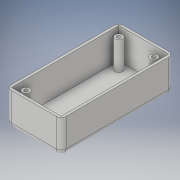
# Autodesk Inventor part: BottomcaseV2
Saved by Autodesk Inventor 2019 (Build 230136000, 136)
## iProperties
Created: 2019-05-05
Part Number: BottomcaseV2
Material: Generic
Document SubType Name: Modeling
Designer: Henry
Density: 1 g/cm^3
Appearance: Default
Author: Henry
Autodesk Inventor part; units mm, degrees
ref_plane "YZ Plane" through (0, 0, 0) normal (1, 0, 0) x (0, 1, 0)
ref_plane "XZ Plane" through (0, 0, 0) normal (0, 1, 0) x (-1, 0, 0)
ref_plane "XY Plane" through (0, 0, 0) normal (0, 0, 1) x (1, 0, 0)
sketch "Sketch1" plane through (0, 0, 0) normal (0, 1, 0) x (-1, 0, 0)
  line L0 (0, 0) -> (40.5, 0)
  line L1 (40.5, 0) -> (40.5, -87.5)
  line L2 (40.5, -87.5) -> (0, -87.5)
  line L3 (0, -87.5) -> (0, 0)
  dimension "d0" = 40.5
  dimension "d1" = 87.5
  constraints: 8 end point, 2 parallel, 1 horizontal, 1 perpendicular
  measures "d0" distance of L1.end L2.end
  measures "d1" distance of L0.end L1.end
extrude "Extrusion1" add sketch "Sketch1" along normal blind 2
sketch "Sketch3" plane through (0, 2, 0) normal (0, 1, 0) x (1, 0, 0)
  line L0 (-40.5, 0) -> (0, 0) projected
  line L1 (-40.5, 0) -> (-34.5, 0)
  line L2 (-34.5, 0) -> (-34.5, 6)
  line L3 (-34.5, 6) -> (-40.5, 6)
  line L4 (-40.5, 6) -> (-40.5, 0)
  circle A0 centre (-34.5, 6) radius 3
  line L5 (-40.5, 87.5) -> (-40.5, 0) projected
  line L6 (-40.5, 87.5) -> (-34.5, 87.5)
  line L7 (-34.5, 87.5) -> (-34.5, 81.5)
  line L8 (-34.5, 81.5) -> (-40.5, 81.5)
  line L9 (-40.5, 81.5) -> (-40.5, 87.5)
  circle A1 centre (-34.5, 81.5) radius 3
  line L10 (0, 0) -> (0, 87.5) projected
  line L11 (0, 87.5) -> (-6, 87.5)
  line L12 (-6, 87.5) -> (-6, 81.5)
  line L13 (-6, 81.5) -> (0, 81.5)
  line L14 (0, 81.5) -> (0, 87.5)
  circle A2 centre (-6, 81.5) radius 3
  dimension "d4" = 6
  dimension "d5" = 6
  dimension "d6" = 6
  dimension "d7" = 6
  dimension "d8" = 6
  dimension "d9" = 6
  dimension "d10" = 6
  dimension "d11" = 6
  dimension "d12" = 6
  constraints: 24 end point, 6 parallel, 3 centre point, 3 coincident, 3 horizontal, 3 perpendicular
  measures "d4" distance of L3.end L2.end
  measures "d5" distance of L2.end L1.end
  measures "d6" diameter of A0
  measures "d7" distance of L7.end L8.end
  measures "d8" distance of L6.end L7.end
  measures "d9" diameter of A1
  measures "d10" distance of L13.end L12.end
  measures "d11" distance of L12.end L11.end
  measures "d12" diameter of A2
extrude "Extrusion2" add sketch "Sketch3" along normal blind 23 contours A0 L3 L2 | L2 L3 A0 | A1 L7 L8 | L8 L7 A1 | A2 L12 L13 | L13 L12 A2
sketch "Sketch4" plane through (-34.5, 25, -6) normal (0, 1, 0) x (1, 0, 0)
  circle A0 centre (0, 0) radius 1.5
  point P0 (34.5, -6)
  dimension "d15" = 3
  constraints: 1 centre point
  measures "d15" diameter of A0
sketch "Sketch5" plane through (-34.5, 25, -81.5) normal (0, 1, 0) x (1, 0, 0)
  circle A0 centre (0, 0) radius 1.5
  point P0 (34.5, -81.5)
  dimension "d16" = 3
  constraints: 1 centre point
  measures "d16" diameter of A0
sketch "Sketch6" plane through (-6, 25, -81.5) normal (0, 1, 0) x (1, 0, 0)
  circle A0 centre (0, 0) radius 1.5
  point P0 (6, -81.5)
  dimension "d17" = 3
  constraints: 1 centre point
  measures "d17" diameter of A0
extrude "Extrusion3" cut sketch "Sketch4" against normal blind 12
extrude "Extrusion4" cut sketch "Sketch5" against normal blind 12
extrude "Extrusion5" cut sketch "Sketch6" against normal blind 12
sketch "Sketch7" plane through (0, 0, 0) normal (0, -1, 0) x (1, 0, 0)
  line L0 (0, 0) -> (0, -87.5) projected
  line L1 (0, 0) -> (2, 0)
  line L2 (2, 0) -> (2, -87.5)
  line L3 (2, -87.5) -> (0, -87.5)
  line L4 (0, -87.5) -> (0, 0)
  line L5 (-40.5, 0) -> (0, 0) projected
  line L6 (-40.5, 0) -> (-42.5, 0)
  line L7 (-42.5, 0) -> (-42.5, -87.5)
  line L8 (-42.5, -87.5) -> (-40.5, -87.5)
  line L9 (-40.5, -87.5) -> (-40.5, 0)
  line L10 (-42.5, -87.5) -> (2, -87.5)
  line L11 (2, -87.5) -> (2, -89.5)
  line L12 (2, -89.5) -> (-42.5, -89.5)
  line L13 (-42.5, -89.5) -> (-42.5, -87.5)
  line L14 (-42.5, 0) -> (2, 0)
  line L15 (2, 0) -> (2, 2)
  line L16 (2, 2) -> (-42.5, 2)
  line L17 (-42.5, 2) -> (-42.5, 0)
  dimension "d24" = 2
  dimension "d25" = 2
  dimension "d26" = 2
  dimension "d27" = 2
  constraints: 32 end point, 8 parallel, 4 horizontal, 4 perpendicular, 1 point on line
  measures "d24" distance of L2.end L3.end
  measures "d25" distance of L8.end L7.end
  measures "d26" distance of L10.end L11.end
  measures "d27" distance of L15.end L14.end
extrude "Extrusion6" add sketch "Sketch7" against normal blind 27 contours L1 L2 L3 L0 | L5 L6 L17 L16 L15 L1 | L3 L11 L12 L13 L8 L10 | L9 L8 L7 L6
fillet "Fillet1" radius 4 8 edges at (2, 13.5, 2) (2, 13.5, -89.5) (-42.5, 13.5, -89.5) (-42.5, 13.5, 2) (-20.25, 0, 2) (-42.5, 0, -43.75) (-20.25, 0, -89.5) (2, 0, -43.75)
body "Solid1"
